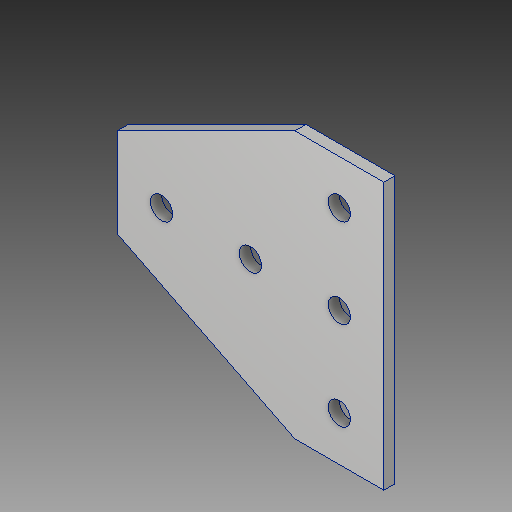
# Autodesk Inventor part: 15102898-16-P-0210
Saved by Autodesk Inventor 2017 (Build 210142000, 142)
## iProperties
Created: 2016-10-03
Part Number: 15102898-16-P-0210
Material: Aluminum 6061
Document SubType Name: Modeling
Designer: gus
Density: 2.7 g/cm^3
Appearance: Aluminum - Flat
Mass: 37.357 g
Surface Area: 98.7677 cm^2
Volume: 13.8359 cm^3
Author: gus
Autodesk Inventor part; units mm, degrees
ref_plane "YZ Plane" through (0, 0, 0) normal (1, 0, 0) x (0, 1, 0)
ref_plane "XZ Plane" through (0, 0, 0) normal (0, 1, 0) x (-1, 0, 0)
ref_plane "XY Plane" through (0, 0, 0) normal (0, 0, 1) x (1, 0, 0)
sketch "Sketch1" plane through (0, 0, 0) normal (0, 0, 1) x (1, 0, 0)
  line L0 (0, 0) -> (0, -76.2)
  line L1 (0, 0) -> (76.2, 0) construction
  line L2 (0, 0) -> (-25.4, 0)
  line L3 (-25.4, 0) -> (-76.2, -25.4)
  line L4 (-76.2, -25.4) -> (-76.2, -50.8)
  line L5 (-76.2, -50.8) -> (-25.4, -76.2)
  line L6 (-25.4, -76.2) -> (0, -76.2)
  circle A0 centre (-12.7, -12.7) radius 3.175
  circle A1 centre (-12.7, -38.1) radius 3.175
  circle A2 centre (-12.7, -63.5) radius 3.175
  circle A3 centre (-38.1, -38.1) radius 3.175
  circle A4 centre (-63.5, -38.1) radius 3.175
  dimension "d0" = 76.2
  dimension "d2" = 25.4
  dimension "d3" = 25.4
  dimension "d4" = 25.4
  dimension "d5" = 76.2
  dimension "d6" = 6.35
  dimension "d7" = 12.7
  dimension "d8" = 12.7
  dimension "d9" = 12.7
  dimension "d10" = 38.1
  dimension "d11" = 25.4
  dimension "d12" = 25.4
  dimension "d13" = 12.7
  dimension "d14" = 12.7
  dimension "d15" = 12.7
  dimension "d16" = 12.7
  constraints: 14 end point, 5 centre point, 4 equal radius, 2 equal length, 2 horizontal, 2 perpendicular, 1 vertical
  measures "d0" distance of L0.start L0.end
  measures "d2" distance of L0.start L2.end
  measures "d3" distance of L5.end L0.end
  measures "d4" distance of L3.end L4.end
  measures "d5" distance between parallel lines of L4 L0
  measures "d6" diameter of A1
  measures "d7" distance from line of L0 A0.centre
  measures "d8" distance from line of L0 A1.centre
  measures "d9" distance from line of A2.centre L0
  measures "d10" distance from line of L0 A3.centre
  measures "d11" distance of A2.centre A1.centre
  measures "d12" distance of A1.centre A0.centre
  measures "d13" distance from line of L2 A0.centre
  measures "d14" vertical distance of L3.end A3.centre
  measures "d15" horizontal distance of L4.end A4.centre
  measures "d16" distance from line of L4 A4.centre
extrude "Extrusion1" add sketch "Sketch1" along normal blind 3.175
body "Solid1"
